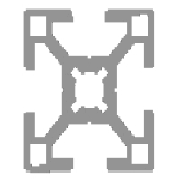
# Autodesk Inventor part: COTS_ARMA_AR3703_30x30_Alu_Extr_00000010
Saved by Autodesk Inventor 2026.1 (Build 301233000, 233)
## iProperties
IsCustomPart: 1
Created: 2016-06-16
Part Number: COTS_ARMA_AR3703_30x30_Alu_Extr_00000010
Material: Aluminium 6061
Description: Profil aluminiowy
Document SubType Name: Modeling
Standard: Bez nazwy
Designer: Andrzej
Language: pl-PL
Size Designation: AR3703 profil 30x30 Frexo
Categories: <MemberInstance><Categories><Category DisplayName="Kształtowniki konstrukcyjne" InternalName="089c4875-fa83-4c05-b084-43b9cc11f5ed" Mnemonic="GRDR"><CategoryParameter DisplayName="Masa na jednostkę długości" InternalName="0bb95a10-148f-4027-a459-38d7b056702a" Mnemonic="shpmass"/><CategoryParameter DisplayName="Powierzchnia przekroju" InternalName="1ff91680-64b0-4202-b9a3-7fd3f94bba3b" Mnemonic="secarea"/><CategoryParameter DisplayName="Promień obrotu (x)" InternalName="25778675-03e9-40c1-b6a8-4a9ed693320d" Mnemonic="gyrradx"/><CategoryParameter DisplayName="Moduł sztywności skrętnej" InternalName="26c1ec35-5026-4c63-ad0a-751cf684a536" Mnemonic="torrigmod"/><CategoryParameter DisplayName="Odległość środka ciężkości X-X" InternalName="26c9bdb8-9c79-4b4f-a92e-8e197583c9c4" Mnemonic="grcendistX"/><CategoryParameter DisplayName="ID elementu typowego" InternalName="340afe4f-75d7-48d3-ab7d-943f3c3da468" Mnemonic="LegacyMemberID"/><CategoryParameter DisplayName="Długość podstawowa" InternalName="42e34263-8f20-4d0e-ad48-bf1385b87c24" Mnemonic="shplen"/><CategoryParameter DisplayName="Moment bezwładności (y)" InternalName="4b9f58ea-bced-460e-81ea-3d29ca5a49e3" Mnemonic="inermomy"/><CategoryParameter DisplayName="Moment bezwładności (x)" InternalName="4cd780bc-73d7-43ac-917a-579e5cbd684d" Mnemonic="inermomx"/><CategoryParameter DisplayName="Niestandardowy punkt podstawowy" InternalName="4f1d1b73-316d-484b-a3df-9cbabb16eb77" Mnemonic="shpBasePoint"/><CategoryParameter DisplayName="Wysokość kształtki" InternalName="50274e7d-5ac0-4796-92cb-c59e54983c67" Mnemonic="shpheig"/><CategoryParameter DisplayName="Moduł wytrzymałości przekroju (y)" InternalName="59eaa5e9-d227-48dc-b6c1-6920f96e0f95" Mnemonic="secmody"/><CategoryParameter DisplayName="Oznaczenie fragmentu" InternalName="5a64d034-428d-49c8-ba32-7619764de20f" Mnemonic="shpdes"/><CategoryParameter DisplayName="Moduł wytrzymałości przekroju (x)" InternalName="72cfad18-cf51-4ed4-aaa7-c6b224f8419f" Mnemonic="secmodx"/><CategoryParameter DisplayName="Moduł wytrzymałości przekroju na skręcanie" InternalName="7c55a8dc-8844-49f9-a867-cc677b30ec9a" Mnemonic="torsecmod"/><CategoryParameter DisplayName="Szerokość kształtki" InternalName="7c717d54-a18f-4666-b4d4-573cce22c62c" Mnemonic="shpwdth"/><CategoryParameter DisplayName="Grubość drugiej kształtki" InternalName="9251a8e1-85fd-4e47-af99-afdb762317d9" Mnemonic="shpthick2"/><CategoryParameter DisplayName="Złącze zatwierdzone" InternalName="9c666724-f362-4ea7-ac62-f6a007de5c69" Mnemonic="shpFGAuto"/><CategoryParameter DisplayName="Odległość środka ciężkości Y-Y" InternalName="bcc4fb17-7af4-436a-8f8c-d0aa3b0248c5" Mnemonic="grcendistY"/><CategoryParameter DisplayName="Promień obrotu (y)" InternalName="bfa18ebe-1636-4dbe-8d42-b263e0b73184" Mnemonic="gyrrady"/><CategoryParameter DisplayName="Grubość kształtki" InternalName="d109cf76-8eb4-42fc-9800-4409734adc67" Mnemonic="shpthick"/><CategoryParameter DisplayName="Współczynnik przesunięcia w wyniku ścinania" InternalName="de4c90c6-aaa8-468f-a335-6737b311b5d3" Mnemonic="shdispc"/><Category DisplayName="Inne" InternalName="f02205ff-2390-476f-921c-0b3185f88e84" Mnemonic="OTHSHP"><CategoryParameter DisplayName="Moment bezwładności (y)" InternalName="044c654e-f649-48ac-84cc-650a29ae31ca" Mnemonic="inermomy"/><CategoryParameter DisplayName="Grubość kształtki" InternalName="12b1a788-9233-48fd-a933-2df8ff42b15f" Mnemonic="shpthick"/><CategoryParameter DisplayName="Masa na jednostkę długości" InternalName="2fd289d6-9394-4d2d-97e6-6659d7d4551d" Mnemonic="shpmass"/><CategoryParameter DisplayName="Promień obrotu (y)" InternalName="743e1dfe-1bba-408b-b985-cf752b207386" Mnemonic="gyrrady"/><CategoryParameter DisplayName="Moduł wytrzymałości przekroju (y)" InternalName="88b8bff9-a616-4028-93d5-ed4f79680d13" Mnemonic="secmody"/><CategoryParameter DisplayName="Powierzchnia przekroju" InternalName="c46ecdf8-b6eb-4db9-8b25-30258930c1e3" Mnemonic="secarea"/><CategoryParameter DisplayName="Moduł wytrzymałości przekroju (x)" InternalName="cac70804-9d39-43bb-be17-56ea1f39a6c2" Mnemonic="secmodx"/><CategoryParameter DisplayName="Moment bezwładności (x)" InternalName="ec6737bc-264f-43ed-b0bd-f6d410c2718d" Mnemonic="inermomx"/><CategoryParameter DisplayName="Promień obrotu (x)" InternalName="ee72c61e-565e-4fd6-b448-66e1e1abcb7e" Mnemonic="gyrradx"/></Category></Category><Category DisplayName="TypDanych" InternalName="23b78d0f-2648-40c6-8793-ca6db495c9e8" Mnemonic="DATATYPE"><CategoryParameter DisplayName="NazwaWyświetlana" InternalName="05415f3d-3907-474b-a020-eb9d644f4cf3" Mnemonic="DISPLAYNAME"/><CategoryParameter DisplayName="Standardowe" InternalName="0c0a119c-1e12-4c84-803f-101930972f5e" Mnemonic="STANDARD"/><CategoryParameter DisplayName="Opis" InternalName="13903e3d-64b1-4950-80da-f627842ea37f" Mnemonic="DESCRIPTION"/><CategoryParameter DisplayName="Oznaczenie" InternalName="2675968c-4ce5-49e0-a4f5-552d29089031" Mnemonic="DESIGNATION"/><CategoryParameter DisplayName="Wiersz domyślny" InternalName="2af9ec52-faaa-4026-b378-f9fa4afca842" Mnemonic="DEFAULTROW"/><CategoryParameter DisplayName="Nazwa folderu" InternalName="3f06958e-8713-4116-9be7-ed6184ecc97b" Mnemonic="FOLDERNAME"/><CategoryParameter DisplayName="Wskazówki do poprawek" InternalName="45a75005-10b1-4dfc-8d6d-dfe629f0b93c" Mnemonic="REVISIONGUID"/><CategoryParameter DisplayName="Nazwa pliku" InternalName="8b46a4cc-9585-4fed-90c3-899f57e09a73" Mnemonic="FILENAME"/><CategoryParameter DisplayName="OrgStd" InternalName="8f5914e1-4693-403f-8ab5-d37768198c9d" Mnemonic="STDSORG"/><CategoryParameter DisplayName="Wersja rodziny" InternalName="914462f6-6e19-4b14-ba84-155b9680b1d0" Mnemonic="FAMILYREVISION"/><CategoryParameter DisplayName="Poprawka standardowa" InternalName="91d5a463-65c2-4fde-b823-3b7fea5e8e17" Mnemonic="STANDARDREVISION"/><CategoryParameter DisplayName="Zmiana elementu" InternalName="a65d44b9-392f-4f4f-857b-e4b3d54996fe" Mnemonic="MEMBERREVISION"/><CategoryParameter DisplayName="FormatKlipu" InternalName="bc51e27b-3422-4e78-93ef-cec197ddf230" Mnemonic="CLIPFORMAT"/><CategoryParameter DisplayName="Producent" InternalName="cd6c7a72-a28a-4e50-99a9-2c7f4e13e5ad" Mnemonic="MANUFACTURER"/><CategoryParameter DisplayName="NazwaWewnętrzna" InternalName="cf1d0246-76d9-4b4a-8305-fa0409afb5c1" Mnemonic="INTERNALNAME"/><CategoryParameter DisplayName="CzyMetryczne" InternalName="e2385c5b-1ea4-4823-96a8-8de651266ec3" Mnemonic="ISMETRIC"/><Category DisplayName="Część" InternalName="c0e0b642-3bcb-4cc8-9e80-f96d35c4afa4" Mnemonic="PART"><CategoryParameter DisplayName="Numer części" InternalName="016b6077-bfbe-49bd-92c9-d8d59c39c941" Mnemonic="PARTNUMBER"/><CategoryParameter DisplayName="Numer katalogowy" InternalName="4dba7c1c-e26c-444e-836c-b08b433409a8" Mnemonic="STOCKNUMBER"/><CategoryParameter DisplayName="Klucz - materiał" InternalName="5c9a8adb-dd2b-4535-b97f-0a94a95fe41f" Mnemonic="MATERIALKEY"/><CategoryParameter DisplayName="Materiał" InternalName="818a152a-d3c3-49ca-80ee-df7d91421b8e" Mnemonic="MATERIAL"/></Category></Category></Categories><FamilyTemplate Id="AR3703 profil 30x30 Frexo"><FamilyTemplateParameters><FamilyTemplateParameter ObjectType="kModelParameterObject" ValueType="xs:double" Id="12" ObjectReferenceKey="Length"/><FamilyTemplateParameter ObjectType="kPartComponentDefinitionObject" ValueType="xs:string" Id="23" SubObjectId="Material"/><FamilyTemplateParameter ObjectType="kPropertyObject" ValueType="xs:string" Id="26" ObjectReferenceKey="{32853F0F-3444-11d1-9E93-0060B03C1CA6}" SubObjectId="5"/><FamilyTemplateParameter ObjectType="kPropertyObject" ValueType="xs:string" Id="27" ObjectReferenceKey="{32853F0F-3444-11d1-9E93-0060B03C1CA6}" SubObjectId="52"/></FamilyTemplateParameters></FamilyTemplate><CategoryParameterMap><ParamToTemplateMap><ParamToTemplate CategoryParameter="//CategoryParameter[@InternalName='cf1d0246-76d9-4b4a-8305-fa0409afb5c1']" ConstantValue="79aeb314-74c3-4d35-89bb-f9897b770a67"/><ParamToTemplate CategoryParameter="//CategoryParameter[@InternalName='45a75005-10b1-4dfc-8d6d-dfe629f0b93c']" ConstantValue="43264b45-992d-42bc-82b9-981101c1b33b"/><ParamToTemplate CategoryParameter="//CategoryParameter[@InternalName='3f06958e-8713-4116-9be7-ed6184ecc97b']" ConstantValue="AR3703 profil 30x30 Frexo"/><ParamToTemplate CategoryParameter="//CategoryParameter[@InternalName='8f5914e1-4693-403f-8ab5-d37768198c9d']" TemplateParameter="17"/><ParamToTemplate CategoryParameter="//CategoryParameter[@InternalName='0c0a119c-1e12-4c84-803f-101930972f5e']" TemplateParameter="18"/><ParamToTemplate CategoryParameter="//CategoryParameter[@InternalName='91d5a463-65c2-4fde-b823-3b7fea5e8e17']" TemplateParameter="19"/><ParamToTemplate CategoryParameter="//CategoryParameter[@InternalName='cd6c7a72-a28a-4e50-99a9-2c7f4e13e5ad']" TemplateParameter="20"/><ParamToTemplate CategoryParameter="//CategoryParameter[@InternalName='13903e3d-64b1-4950-80da-f627842ea37f']" ConstantValue="Profil aluminiowy"/><ParamToTemplate CategoryParameter="//CategoryParameter[@InternalName='05415f3d-3907-474b-a020-eb9d644f4cf3']" ConstantValue="AR3703 profil 30x30 Frexo"/><ParamToTemplate CategoryParameter="//CategoryParameter[@InternalName='914462f6-6e19-4b14-ba84-155b9680b1d0']" ConstantValue="11"/><ParamToTemplate CategoryParameter="//CategoryParameter[@InternalName='bc51e27b-3422-4e78-93ef-cec197ddf230']" ConstantValue="CF_INVENTOR.STDPARTS"/><ParamToTemplate CategoryParameter="//CategoryParameter[@InternalName='e2385c5b-1ea4-4823-96a8-8de651266ec3']" ConstantValue="true"/><ParamToTemplate CategoryParameter="//CategoryParameter[@InternalName='2af9ec52-faaa-4026-b378-f9fa4afca842']" ConstantValue="1"/><ParamToTemplate CategoryParameter="//CategoryParameter[@InternalName='9c666724-f362-4ea7-ac62-f6a007de5c69']" ConstantValue="1"/><ParamToTemplate CategoryParameter="//CategoryParameter[@InternalName='8b46a4cc-9585-4fed-90c3-899f57e09a73']" ConstantValue="AR3703 profil 30x30 Frexo"/><ParamToTemplate CategoryParameter="//CategoryParameter[@InternalName='a65d44b9-392f-4f4f-857b-e4b3d54996fe']" ConstantValue="2e95c903-b951-4fd9-b45f-d5ada82a64a5"/><ParamToTemplate CategoryParameter="//CategoryParameter[@InternalName='a65d44b9-392f-4f4f-857b-e4b3d54996fe']" ConstantValue="2e95c903-b951-4fd9-b45f-d5ada82a64a5"/><ParamToTemplate CategoryParameter="//CategoryParameter[@InternalName='2675968c-4ce5-49e0-a4f5-552d29089031']" TemplateParameter="27"/><ParamToTemplate CategoryParameter="//CategoryParameter[@InternalName='42e34263-8f20-4d0e-ad48-bf1385b87c24']" TemplateParameter="12"/><ParamToTemplate CategoryParameter="//CategoryParameter[@InternalName='818a152a-d3c3-49ca-80ee-df7d91421b8e']" TemplateParameter="23"/><ParamToTemplate CategoryParameter="//CategoryParameter[@InternalName='016b6077-bfbe-49bd-92c9-d8d59c39c941']" TemplateParameter="26"/></ParamToTemplateMap></CategoryParameterMap></MemberInstance>
Density: 2.7 g/cm^3
Appearance: Anodized - Light Gray
Mass: 403.032 g
Surface Area: 1761.55 cm^2
Volume: 149.271 cm^3
_CCFamilyDisplayName: AR3703 profil 30x30 Frexo - Profil aluminiowy
_FrameMemberDoc: Frame Member File
_Version: 15.0.0
_GetPNFromCC: 1
G_L: 502,000 mm
G_W: 30,000 mm
G_H: 30,000 mm
+94B9E9C2-02E4-4FB9-8258-5535166FFC77+CUTDETAIL1: Wytnij
+AFEB632A-2FBC-4D66-A86B-28FDF740D37E+CUTDETAIL2: Wytnij
Author: Andrzej
Autodesk Inventor part; units mm, degrees
ref_plane "Płaszczyzna początkowa" through (0, 0, 15) normal (0, 0, 1) x (1, 0, 0)
ref_plane "Płaszczyzna końcowa" through (0, 0, 517) normal (0, 0, 1) x (1, 0, 0)
sketch "Szkic" plane through (0, 0, 0) normal (0, 0, 1) x (1, 0, 0)
  line L0 (1.7751, -3.1893) -> (3.1172, -4.5314)
  arc A0 (-1.7751, -3.1893) -> (1.7751, -3.1893) centre (0, 0) ccw
  line L1 (-3.1172, -4.5314) -> (-1.7751, -3.1893)
  arc A1 (-4.5314, -3.1172) -> (-3.1172, -4.5314) centre (0, 0) ccw
  line L2 (-3.1893, -1.7751) -> (-4.5314, -3.1172)
  arc A2 (-3.1893, 1.7751) -> (-3.1893, -1.7751) centre (0, 0) ccw
  line L3 (-4.5314, 3.1172) -> (-3.1893, 1.7751)
  arc A3 (-3.1172, 4.5314) -> (-4.5314, 3.1172) centre (0, 0) ccw
  line L4 (-1.7751, 3.1893) -> (-3.1172, 4.5314)
  arc A4 (1.7751, 3.1893) -> (-1.7751, 3.1893) centre (0, 0) ccw
  line L5 (3.1172, 4.5314) -> (1.7751, 3.1893)
  arc A5 (4.5314, 3.1172) -> (3.1172, 4.5314) centre (0, 0) ccw
  line L6 (3.1893, 1.7751) -> (4.5314, 3.1172)
  arc A6 (3.1893, -1.7751) -> (3.1893, 1.7751) centre (0, 0) ccw
  line L7 (4.5314, -3.1172) -> (3.1893, -1.7751)
  arc A7 (3.1172, -4.5314) -> (4.5314, -3.1172) centre (0, 0) ccw
  line L8 (14, -13.5) -> (14, -9.9)
  arc A8 (13.5, -14) -> (14, -13.5) centre (13.5, -13.5) ccw
  line L9 (9.9, -14) -> (13.5, -14)
  line L10 (9.9, -9.9) -> (9.9, -14)
  line L11 (14, -9.9) -> (9.9, -9.9)
  line L12 (-9.9, -9.9) -> (-14, -9.9)
  line L13 (-9.9, -14) -> (-9.9, -9.9)
  line L14 (-13.5, -14) -> (-9.9, -14)
  arc A9 (-14, -13.5) -> (-13.5, -14) centre (-13.5, -13.5) ccw
  line L15 (-14, -9.9) -> (-14, -13.5)
  line L16 (14, 9.9) -> (14, 13.5)
  line L17 (9.9, 9.9) -> (14, 9.9)
  line L18 (9.9, 14) -> (9.9, 9.9)
  line L19 (13.5, 14) -> (9.9, 14)
  arc A10 (14, 13.5) -> (13.5, 14) centre (13.5, 13.5) ccw
  line L20 (-14, 9.9) -> (-9.9, 9.9)
  line L21 (-14, 13.5) -> (-14, 9.9)
  arc A11 (-13.5, 14) -> (-14, 13.5) centre (-13.5, 13.5) ccw
  line L22 (-9.9, 14) -> (-13.5, 14)
  line L23 (-9.9, 9.9) -> (-9.9, 14)
  line L24 (13.5, -15) -> (4.5, -15)
  arc A12 (13.5, -15) -> (15, -13.5) centre (13.5, -13.5) ccw
  line L25 (15, -4.5) -> (15, -13.5)
  line L26 (14.5, -4.5) -> (15, -4.5)
  line L27 (14.5, -4) -> (14.5, -4.5)
  line L28 (12.9, -4) -> (14.5, -4)
  arc A13 (12.9, -4) -> (12.8, -4.1) centre (12.9, -4.1) ccw
  line L29 (12.8, -8.6) -> (12.8, -4.1)
  arc A14 (12.5, -8.9) -> (12.8, -8.6) centre (12.5, -8.6) ccw
  line L30 (10.5799, -8.9) -> (12.5, -8.9)
  arc A15 (10.3678, -8.8121) -> (10.5799, -8.9) centre (10.5799, -8.6) ccw
  line L31 (6.1179, -4.5622) -> (10.3678, -8.8121)
  arc A16 (6.03, -4.3501) -> (6.1179, -4.5622) centre (6.33, -4.3501) ccw
  line L32 (6.03, -0.5) -> (6.03, -4.3501)
  line L33 (5.53, 0) -> (6.03, -0.5)
  line L34 (6.03, 0.5) -> (5.53, 0)
  line L35 (6.03, 4.3501) -> (6.03, 0.5)
  arc A17 (6.1179, 4.5622) -> (6.03, 4.3501) centre (6.33, 4.3501) ccw
  line L36 (10.3678, 8.8121) -> (6.1179, 4.5622)
  arc A18 (10.5799, 8.9) -> (10.3678, 8.8121) centre (10.5799, 8.6) ccw
  line L37 (12.5, 8.9) -> (10.5799, 8.9)
  arc A19 (12.8, 8.6) -> (12.5, 8.9) centre (12.5, 8.6) ccw
  line L38 (12.8, 4.1) -> (12.8, 8.6)
  arc A20 (12.8, 4.1) -> (12.9, 4) centre (12.9, 4.1) ccw
  line L39 (14.5, 4) -> (12.9, 4)
  line L40 (14.5, 4.5) -> (14.5, 4)
  line L41 (15, 4.5) -> (14.5, 4.5)
  line L42 (15, 13.5) -> (15, 4.5)
  arc A21 (15, 13.5) -> (13.5, 15) centre (13.5, 13.5) ccw
  line L43 (4.5, 15) -> (13.5, 15)
  line L44 (4.5, 14.5) -> (4.5, 15)
  line L45 (4, 14.5) -> (4.5, 14.5)
  line L46 (4, 12.9) -> (4, 14.5)
  arc A22 (4, 12.9) -> (4.1, 12.8) centre (4.1, 12.9) ccw
  line L47 (8.6, 12.8) -> (4.1, 12.8)
  arc A23 (8.9, 12.5) -> (8.6, 12.8) centre (8.6, 12.5) ccw
  line L48 (8.9, 10.5799) -> (8.9, 12.5)
  arc A24 (8.8121, 10.3678) -> (8.9, 10.5799) centre (8.6, 10.5799) ccw
  line L49 (4.5622, 6.1179) -> (8.8121, 10.3678)
  arc A25 (4.3501, 6.03) -> (4.5622, 6.1179) centre (4.3501, 6.33) ccw
  line L50 (0.5, 6.03) -> (4.3501, 6.03)
  line L51 (0, 5.53) -> (0.5, 6.03)
  line L52 (-0.5, 6.03) -> (0, 5.53)
  line L53 (-4.3501, 6.03) -> (-0.5, 6.03)
  arc A26 (-4.5622, 6.1179) -> (-4.3501, 6.03) centre (-4.3501, 6.33) ccw
  line L54 (-8.8121, 10.3678) -> (-4.5622, 6.1179)
  arc A27 (-8.9, 10.5799) -> (-8.8121, 10.3678) centre (-8.6, 10.5799) ccw
  line L55 (-8.9, 12.5) -> (-8.9, 10.5799)
  arc A28 (-8.6, 12.8) -> (-8.9, 12.5) centre (-8.6, 12.5) ccw
  line L56 (-4.1, 12.8) -> (-8.6, 12.8)
  arc A29 (-4.1, 12.8) -> (-4, 12.9) centre (-4.1, 12.9) ccw
  line L57 (-4, 14.5) -> (-4, 12.9)
  line L58 (-4.5, 14.5) -> (-4, 14.5)
  line L59 (-4.5, 15) -> (-4.5, 14.5)
  line L60 (-13.5, 15) -> (-4.5, 15)
  arc A30 (-13.5, 15) -> (-15, 13.5) centre (-13.5, 13.5) ccw
  line L61 (-15, 4.5) -> (-15, 13.5)
  line L62 (-14.5, 4.5) -> (-15, 4.5)
  line L63 (-14.5, 4) -> (-14.5, 4.5)
  line L64 (-12.9, 4) -> (-14.5, 4)
  arc A31 (-12.9, 4) -> (-12.8, 4.1) centre (-12.9, 4.1) ccw
  line L65 (-12.8, 8.6) -> (-12.8, 4.1)
  arc A32 (-12.5, 8.9) -> (-12.8, 8.6) centre (-12.5, 8.6) ccw
  line L66 (-10.5799, 8.9) -> (-12.5, 8.9)
  arc A33 (-10.3678, 8.8121) -> (-10.5799, 8.9) centre (-10.5799, 8.6) ccw
  line L67 (-6.1179, 4.5622) -> (-10.3678, 8.8121)
  arc A34 (-6.03, 4.3501) -> (-6.1179, 4.5622) centre (-6.33, 4.3501) ccw
  line L68 (-6.03, 0.5) -> (-6.03, 4.3501)
  line L69 (-5.53, 0) -> (-6.03, 0.5)
  line L70 (-6.03, -0.5) -> (-5.53, 0)
  line L71 (-6.03, -4.3501) -> (-6.03, -0.5)
  arc A35 (-6.1179, -4.5622) -> (-6.03, -4.3501) centre (-6.33, -4.3501) ccw
  line L72 (-10.3678, -8.8121) -> (-6.1179, -4.5622)
  arc A36 (-10.5799, -8.9) -> (-10.3678, -8.8121) centre (-10.5799, -8.6) ccw
  line L73 (-12.5, -8.9) -> (-10.5799, -8.9)
  arc A37 (-12.8, -8.6) -> (-12.5, -8.9) centre (-12.5, -8.6) ccw
  line L74 (-12.8, -4.1) -> (-12.8, -8.6)
  arc A38 (-12.8, -4.1) -> (-12.9, -4) centre (-12.9, -4.1) ccw
  line L75 (-14.5, -4) -> (-12.9, -4)
  line L76 (-14.5, -4.5) -> (-14.5, -4)
  line L77 (-15, -4.5) -> (-14.5, -4.5)
  line L78 (-15, -13.5) -> (-15, -4.5)
  arc A39 (-15, -13.5) -> (-13.5, -15) centre (-13.5, -13.5) ccw
  line L79 (-4.5, -15) -> (-13.5, -15)
  line L80 (-4.5, -14.5) -> (-4.5, -15)
  line L81 (-4, -14.5) -> (-4.5, -14.5)
  line L82 (-4, -12.9) -> (-4, -14.5)
  arc A40 (-4, -12.9) -> (-4.1, -12.8) centre (-4.1, -12.9) ccw
  line L83 (-8.6, -12.8) -> (-4.1, -12.8)
  arc A41 (-8.9, -12.5) -> (-8.6, -12.8) centre (-8.6, -12.5) ccw
  line L84 (-8.9, -10.5799) -> (-8.9, -12.5)
  arc A42 (-8.8121, -10.3678) -> (-8.9, -10.5799) centre (-8.6, -10.5799) ccw
  line L85 (-4.5622, -6.1179) -> (-8.8121, -10.3678)
  arc A43 (-4.3501, -6.03) -> (-4.5622, -6.1179) centre (-4.3501, -6.33) ccw
  line L86 (-0.5, -6.03) -> (-4.3501, -6.03)
  line L87 (0, -5.53) -> (-0.5, -6.03)
  line L88 (0.5, -6.03) -> (0, -5.53)
  line L89 (4.3501, -6.03) -> (0.5, -6.03)
  arc A44 (4.5622, -6.1179) -> (4.3501, -6.03) centre (4.3501, -6.33) ccw
  line L90 (8.8121, -10.3678) -> (4.5622, -6.1179)
  arc A45 (8.9, -10.5799) -> (8.8121, -10.3678) centre (8.6, -10.5799) ccw
  line L91 (8.9, -12.5) -> (8.9, -10.5799)
  arc A46 (8.6, -12.8) -> (8.9, -12.5) centre (8.6, -12.5) ccw
  line L92 (4.1, -12.8) -> (8.6, -12.8)
  arc A47 (4.1, -12.8) -> (4, -12.9) centre (4.1, -12.9) ccw
  line L93 (4, -14.5) -> (4, -12.9)
  line L94 (4.5, -14.5) -> (4, -14.5)
  line L95 (4.5, -15) -> (4.5, -14.5)
  point P0 (15, -15)
  constraints: 192 end point, 96 point on circle, 48 centre point
extrude "Bryła" add sketch "Szkic" along normal up to surface (502 mm away) from surface at 15
sketch "Szkic2" plane through (0, 0, 0) normal (0, 0, 1) x (1, 0, 0)
  line L0 (0, 0) -> (10, 0)
ref_plane "Płaszczyzna konstrukcyjna3" through (0, 0, 0) normal (0, -1, 0) x (1, 0, 0)
sketch "Szkic3" plane through (0, 0, 0) normal (0, -1, 0) x (1, 0, 0)
  line L0 (-2, 15) -> (12, 15)
  line L1 (-2, 517) -> (12, 517)
  dimension "d7" = 502
  measures "d7" distance between parallel lines of L0 L1
ref_plane "Płaszczyzna konstrukcyjna4" through (4.5, -430, 15) normal (0, 0, -1) x (-1, 0, 0)
split "Podział1" plane through (4.5, -430, 15) removes the side toward (0, 0, -1)
ref_plane "Płaszczyzna konstrukcyjna5" through (13.5, -475, 517) normal (0, 0, 1) x (1, 0, 0)
split "Podział2" plane through (13.5, -475, 517) removes the side toward (0, 0, 1)
equation "\"G_OFFSET_START\" = -15"
equation "\"G_OFFSET_END\" = -15"
equation "\"d2\" = -G_OFFSET_START"
equation "\"d3\" = Length + G_OFFSET_END"
equation "\"G_L\" = d7"
equation "\"Length\" = 532"
